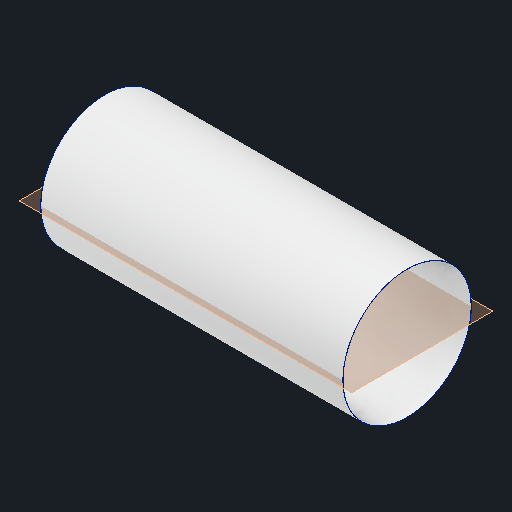
# Autodesk Inventor part: Pressure Vessel, Single Part
Saved by Autodesk Inventor 2026.2 (Build 302298000, 298)
## iProperties
Created: 2025-10-25
Part Number: Pressure Vessel, Single Part
Material: Aluminum 6061
Document SubType Name: Modeling
Designer: Brandon Portillo
Density: 2.7 g/cm^3
Appearance: Aluminum - Flat
Author: Brandon Portillo
Autodesk Inventor part; units mm, degrees
ref_plane "YZ Plane" through (0, 0, 0) normal (1, 0, 0) x (0, 1, 0)
ref_plane "XY Plane" through (0, 0, 0) normal (0, 0, 1) x (1, 0, 0)
sketch "Sketch1" plane through (0, 0, 0) normal (1, 0, 0) x (0, 1, 0)
  circle A0 centre (0, 0) radius 2125
  dimension "d0" = 4250
  constraints: 1 centre point, 1 coincident
  measures "d0" diameter of A0
extrude "Extrusion1" add sketch "Sketch1" against normal blind 10000
shell "Shell1" thickness 5 removed faces 2 at (0, -479.1257, -442.9355) at (-10000, -479.1257, -442.9355)
body "Solid1"
